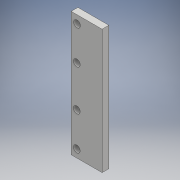
# Autodesk Inventor part: soporte
Saved by Autodesk Inventor 2018 (Build 220112000, 112)
## iProperties
Created: 2018-05-25
Part Number: soporte
Material: Generic
Document SubType Name: Modeling
Designer: vigus
Density: 1 g/cm^3
Appearance: Default
Author: vigus
Autodesk Inventor part; units mm, degrees
ref_plane "YZ Plane" through (0, 0, 0) normal (1, 0, 0) x (0, 1, 0)
ref_plane "XZ Plane" through (0, 0, 0) normal (0, 1, 0) x (-1, 0, 0)
ref_plane "XY Plane" through (0, 0, 0) normal (0, 0, 1) x (1, 0, 0)
sketch "Sketch1" plane through (0, 0, 0) normal (0, 1, 0) x (-1, 0, 0)
  line L0 (8.4467, 22.8129) -> (-5.2472, 22.8129)
  line L1 (-5.2472, 22.8129) -> (-5.2472, -32.1871)
  line L2 (-5.2472, -32.1871) -> (8.4467, -32.1871)
  line L3 (8.4467, -32.1871) -> (8.4467, 22.8129)
  circle A0 centre (5.8231, 19.3129) radius 1.5
  circle A1 centre (5.932, 4.3133) radius 1.5
  circle A2 centre (5.932, -28.6871) radius 1.5
  circle A3 centre (5.932, -13.6871) radius 1.5
  point P0 (0, 0)
  dimension "d0" = 3
  dimension "d1" = 3
  dimension "d2" = 15
  dimension "d3" = 55
  dimension "d4" = 3
  dimension "d5" = 3
  dimension "d6" = 15
  dimension "d7" = 3.5
  dimension "d8" = 3.5
  constraints: 8 end point, 4 centre point, 2 parallel, 1 horizontal, 1 perpendicular
  measures "d0" diameter of A0
  measures "d1" diameter of A1
  measures "d2" distance of A0.centre A1.centre
  measures "d3" distance of L2.end L0.start
  measures "d4" diameter of A2
  measures "d5" diameter of A3
  measures "d6" distance of A3.centre A2.centre
  measures "d7" distance from line of L0 A0.centre
  measures "d8" distance from line of L2 A2.centre
extrude "Extrusion1" add sketch "Sketch1" along normal blind 3
body "Solid1"
